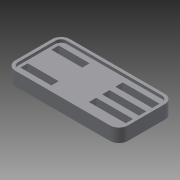
# Autodesk Inventor part: PlugFront
Saved by Autodesk Inventor 2014 SP1 (Build 180222100, 222)
## iProperties
Created: 2014-04-04
Part Number: PlugFront
Material: Generic
Document SubType Name: Modeling
Designer: patrigg
Density: 1 g/cm^3
Appearance: Default
Author: patrigg
Autodesk Inventor part; units mm, degrees
ref_plane "YZ Plane" through (0, 0, 0) normal (1, 0, 0) x (0, 1, 0)
ref_plane "XZ Plane" through (0, 0, 0) normal (0, 1, 0) x (-1, 0, 0)
ref_plane "XY Plane" through (0, 0, 0) normal (0, 0, 1) x (1, 0, 0)
sketch "Sketch1" plane through (0, 0, 0) normal (0, 0, 1) x (1, 0, 0)
  line L0 (0, 0) -> (38.25, 0)
  line L1 (38.25, 0) -> (38.25, 18.6)
  line L2 (38.25, 18.6) -> (0, 18.6)
  line L3 (0, 18.6) -> (0, 0)
  dimension "d0" = 38.25
  dimension "d1" = 18.6
  constraints: 8 end point, 2 parallel, 1 horizontal, 1 perpendicular
  measures "d0" distance between parallel lines of L1 L3
  measures "d1" distance between parallel lines of L0 L2
extrude "Extrusion1" add sketch "Sketch1" along normal blind 1
sketch "Sketch2" plane through (0, 0, 1) normal (0, 0, 1) x (1, 0, 0)
  line L0 (0, 0) -> (38.25, 0) projected
  line L1 (38.25, 0) -> (38.25, 18.6) projected
  line L2 (38.25, 18.6) -> (0, 18.6) projected
  line L3 (0, 18.6) -> (0, 0) projected
  line L4 (2, 16.6) -> (36.25, 16.6) construction
  line L5 (36.25, 16.6) -> (36.25, 2) construction
  line L6 (36.25, 2) -> (2, 2) construction
  line L7 (2, 2) -> (2, 16.6) construction
  line L8 (12.5, 13.3) -> (2, 13.3)
  line L9 (2, 13.3) -> (2, 15.8)
  line L10 (2, 15.8) -> (12.5, 15.8)
  line L11 (12.5, 15.8) -> (12.5, 13.3)
  line L12 (12.5, 2.8) -> (2, 2.8)
  line L13 (2, 2.8) -> (2, 5.3)
  line L14 (2, 5.3) -> (12.5, 5.3)
  line L15 (12.5, 5.3) -> (12.5, 2.8)
  line L16 (23.75, 13.3) -> (36.25, 13.3)
  line L17 (36.25, 13.3) -> (36.25, 15.8)
  line L18 (36.25, 15.8) -> (23.75, 15.8)
  line L19 (23.75, 15.8) -> (23.75, 13.3)
  line L20 (23.75, 8.8) -> (36.25, 8.8)
  line L21 (36.25, 8.8) -> (36.25, 11.3)
  line L22 (36.25, 11.3) -> (23.75, 11.3)
  line L23 (23.75, 11.3) -> (23.75, 8.8)
  line L24 (23.75, 4.3) -> (36.25, 4.3)
  line L25 (36.25, 4.3) -> (36.25, 6.8)
  line L26 (36.25, 6.8) -> (23.75, 6.8)
  line L27 (23.75, 6.8) -> (23.75, 4.3)
  line L28 (2, 2.8) -> (36.25, 2.8) construction
  line L29 (2, 15.8) -> (36.25, 15.8) construction
  line L30 (17.9229, 10.05) -> (35.2346, 10.05) construction
  line L31 (23.75, 15.8) -> (23.75, 2.8) construction
  point P0 (23.75, 10.05)
  dimension "d4" = 2
  dimension "d5" = 2
  dimension "d6" = 2
  dimension "d7" = 2
  dimension "d8" = 0.8
  dimension "d9" = 0.8
  dimension "d10" = 2.5
  dimension "d12" = 10.5
  dimension "d17" = 12.5
  dimension "d20" = 4
  dimension "d21" = 21.75
  constraints: 56 end point, 14 parallel, 8 collinear, 8 perpendicular, 7 equal length, 7 point on line, 6 horizontal, 1 midpoint, 1 other
  measures "d4" distance between parallel lines of L2 L4
  measures "d5" distance between parallel lines of L0 L6
  measures "d6" distance between parallel lines of L3 L7
  measures "d7" distance between parallel lines of L1 L5
  measures "d8" distance between parallel lines of L29 L4
  measures "d9" distance between parallel lines of L28 L6
  measures "d10" distance between parallel lines of L8 L29
  measures "d12" distance between parallel lines of L11 L9
  measures "d17" distance between parallel lines of L17 L19
  measures "d20" distance between parallel lines of L28 L26
  measures "d21" distance between parallel lines of L31 L7
extrude "Extrusion2" add sketch "Sketch2" along normal blind 2.55
sketch "Sketch3" plane through (0, 0, 1) normal (0, 0, 1) x (1, 0, 0)
  line L0 (2, 14.05) -> (12.5, 14.05)
  line L1 (12.5, 14.05) -> (12.5, 15.05)
  line L2 (12.5, 15.05) -> (2, 15.05)
  line L3 (2, 15.05) -> (2, 14.05)
  line L4 (2, 14.05) -> (12.5, 15.05) construction
  line L5 (12.5, 14.05) -> (2, 15.05) construction
  line L6 (2, 13.3) -> (2, 15.8) projected
  line L7 (2, 15.8) -> (12.5, 15.8) projected
  point P0 (0, 0)
  point P1 (7.25, 14.55)
  point P2 (7.25, 14.55)
  point P3 (2, 14.55)
  point P4 (7.25, 14.55)
  point P5 (7.25, 15.8)
  dimension "d24" = 1
  constraints: 12 end point, 6 midpoint, 2 parallel, 1 collinear, 1 horizontal, 1 horizontal alignment, 1 perpendicular, 1 vertical alignment
  measures "d24" distance between parallel lines of L0 L2
extrude "Extrusion3" cut sketch "Sketch3" against normal up to next
sketch "Sketch4" plane through (0, 0, 1) normal (0, 0, 1) x (1, 0, 0)
  line L0 (23.75, 14.05) -> (36.25, 14.05)
  line L1 (36.25, 14.05) -> (36.25, 15.05)
  line L2 (36.25, 15.05) -> (23.75, 15.05)
  line L3 (23.75, 15.05) -> (23.75, 14.05)
  line L4 (23.75, 14.05) -> (36.25, 15.05) construction
  line L5 (36.25, 14.05) -> (23.75, 15.05) construction
  line L6 (23.75, 15.8) -> (36.25, 15.8) projected
  line L7 (23.75, 13.3) -> (23.75, 15.8) projected
  point P0 (0, 0)
  point P1 (30, 14.55)
  point P2 (30, 14.55)
  point P3 (30, 15.8)
  point P4 (30, 14.55)
  point P5 (23.75, 14.55)
  dimension "d27" = 1
  constraints: 12 end point, 6 midpoint, 2 parallel, 1 collinear, 1 horizontal, 1 horizontal alignment, 1 perpendicular, 1 vertical alignment
  measures "d27" distance between parallel lines of L0 L2
extrude "Extrusion4" cut sketch "Sketch4" against normal up to next
sketch "Sketch5" plane through (0, 0, 1) normal (0, 0, 1) x (1, 0, 0)
  line L0 (2, 4.55) -> (12.5, 4.55)
  line L1 (12.5, 4.55) -> (12.5, 3.55)
  line L2 (12.5, 3.55) -> (2, 3.55)
  line L3 (2, 3.55) -> (2, 4.55)
  line L4 (2, 4.55) -> (12.5, 3.55) construction
  line L5 (12.5, 4.55) -> (2, 3.55) construction
  line L6 (2, 5.3) -> (12.5, 5.3) projected
  line L7 (2, 2.8) -> (2, 5.3) projected
  point P0 (0, 0)
  point P1 (7.25, 4.05)
  point P2 (7.25, 4.05)
  point P3 (7.25, 5.3)
  point P4 (7.25, 4.05)
  point P5 (2, 4.05)
  dimension "d30" = 1
  constraints: 12 end point, 6 midpoint, 2 parallel, 1 collinear, 1 horizontal, 1 horizontal alignment, 1 perpendicular, 1 vertical alignment
  measures "d30" distance between parallel lines of L2 L0
extrude "Extrusion5" cut sketch "Sketch5" against normal up to next
sketch "Sketch6" plane through (0, 0, 1) normal (0, 0, 1) x (1, 0, 0)
  line L0 (23.75, 10.55) -> (36.25, 10.55)
  line L1 (36.25, 10.55) -> (36.25, 9.55)
  line L2 (36.25, 9.55) -> (23.75, 9.55)
  line L3 (23.75, 9.55) -> (23.75, 10.55)
  line L4 (23.75, 10.55) -> (36.25, 9.55) construction
  line L5 (36.25, 10.55) -> (23.75, 9.55) construction
  line L6 (23.75, 11.3) -> (36.25, 11.3) projected
  line L7 (23.75, 8.8) -> (23.75, 11.3) projected
  point P0 (0, 0)
  point P1 (30, 10.05)
  point P2 (30, 10.05)
  point P3 (30, 11.3)
  point P4 (30, 10.05)
  point P5 (23.75, 10.05)
  dimension "d33" = 1
  constraints: 12 end point, 6 midpoint, 2 parallel, 1 collinear, 1 horizontal, 1 horizontal alignment, 1 perpendicular, 1 vertical alignment
  measures "d33" distance between parallel lines of L2 L0
extrude "Extrusion6" cut sketch "Sketch6" against normal up to next
sketch "Sketch7" plane through (0, 0, 1) normal (0, 0, 1) x (1, 0, 0)
  line L0 (23.75, 5.05) -> (36.25, 5.05)
  line L1 (36.25, 5.05) -> (36.25, 6.05)
  line L2 (36.25, 6.05) -> (23.75, 6.05)
  line L3 (23.75, 6.05) -> (23.75, 5.05)
  line L4 (23.75, 5.05) -> (36.25, 6.05) construction
  line L5 (36.25, 5.05) -> (23.75, 6.05) construction
  line L6 (23.75, 4.3) -> (23.75, 6.8) projected
  line L7 (23.75, 6.8) -> (36.25, 6.8) projected
  point P0 (0, 0)
  point P1 (30, 5.55)
  point P2 (30, 5.55)
  point P3 (23.75, 5.55)
  point P4 (30, 5.55)
  point P5 (30, 6.8)
  dimension "d36" = 1
  constraints: 12 end point, 6 midpoint, 2 parallel, 1 collinear, 1 horizontal, 1 horizontal alignment, 1 perpendicular, 1 vertical alignment
  measures "d36" distance between parallel lines of L0 L2
extrude "Extrusion7" cut sketch "Sketch7" against normal up to next
fillet "Fillet1" radius 3 4 edges at (0, 0, 1.775) (38.25, 0, 1.775) (0, 18.6, 1.775) (38.25, 18.6, 1.775)
sketch "Sketch8" plane through (0, 0, 0) normal (0, 0, -1) x (-1, 0, 0)
  line L0 (-2, 15.05) -> (-2, 14.05) projected
  line L1 (0, 0) -> (-38.25, 0) projected
  line L2 (0, 18.6) -> (0, 0) projected
  line L3 (-38.25, 18.6) -> (0, 18.6) projected
  line L4 (-38.25, 0) -> (-38.25, 18.6) projected
  line L5 (-2, 18.6) -> (-2, 0)
  constraints: 2 end point, 2 point on line, 1 collinear, 1 parallel
extrude "Extrusion8" cut sketch "Sketch8" against normal blind 2 contours L5 L3 L2 L1 L0
lip "Lip1" kind lip height 1 width 1 edges at (19.125, 0, 3.55) (37.3713, 0.8787, 3.55) (38.25, 9.3, 3.55) (37.3713, 17.7213, 3.55) (19.125, 18.6, 3.55) (0.8787, 17.7213, 3.55) (0, 9.3, 3.55) (0.8787, 0.8787, 3.55) guide face at (20.6667, 17.6667, 3.55)
body "Solid1"
